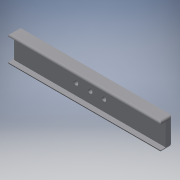
# Autodesk Inventor part: Chain_support
Saved by Autodesk Inventor 2019.3 (Build 233278000, 278)
## iProperties
Created: 2020-09-24
Part Number: Chain_support
Material: Generisch
Document SubType Name: Modeling
Designer: Nicolas Frick
Density: 1 g/cm^3
Appearance: Vorgabe
Author: Nicolas Frick
Autodesk Inventor part; units mm, degrees
ref_plane "YZ Plane" through (0, 0, 0) normal (1, 0, 0) x (0, 1, 0)
ref_plane "XZ Plane" through (0, 0, 0) normal (0, 1, 0) x (-1, 0, 0)
ref_plane "XY Plane" through (0, 0, 0) normal (0, 0, 1) x (1, 0, 0)
sketch "Skizze1" plane through (0, 0, 0) normal (0, 0, 1) x (1, 0, 0)
  line L0 (-23.9848, 119.7892) -> (-23.9848, -119.7892) construction
  line L1 (-23.9848, -119.7892) -> (23.9848, -119.7892) construction
  line L2 (23.9848, -119.7892) -> (23.9848, 119.7892) construction
  line L3 (23.9848, 119.7892) -> (-23.9848, 119.7892) construction
  line L4 (-23.9848, 119.7892) -> (-23.9848, -119.7892) construction
  line L5 (71.859, -124.7444) -> (-78.141, -124.7444)
  line L6 (-78.141, -124.7444) -> (-78.141, -98.7444)
  line L7 (-78.141, -98.7444) -> (71.859, -98.7444)
  line L8 (71.859, -98.7444) -> (71.859, -124.7444)
  circle A0 centre (-16.2025, -111.7444) radius 2.25
  circle A1 centre (11.1538, -111.7444) radius 2.25
  circle A2 centre (-2.2951, -111.7444) radius 2.25
  point P0 (0, 0)
  dimension "d0" = 150
  dimension "d1" = 26
  dimension "d2" = 4.5
  dimension "d3" = 4.5
  dimension "d4" = 4.5
  constraints: 8 end point, 3 centre point, 2 parallel, 1 horizontal, 1 perpendicular
  measures "d0" distance of L6.end L7.end
  measures "d1" distance of L5.end L6.end
  measures "d2" diameter of A0
  measures "d3" diameter of A1
  measures "d4" diameter of A2
ref_plane "Arbeitsebene1" through (175.4546, -108.6892, 6.4137) normal (0, 0, -1) x (0, 1, 0)
extrude "Extrusion1" add sketch "Skizze1" along normal up to surface (6.4137 mm away)
sketch "Skizze3" plane through (-78.141, -124.7444, 6.4137) normal (0, 0, 1) x (1, 0, 0)
  circle A0 centre (75.8459, 13) radius 2.25 construction
  circle A1 centre (89.2948, 13) radius 2.25 construction
  circle A2 centre (61.9385, 13) radius 2.25 construction
  line L0 (0, 26) -> (0, 0) construction
  line L1 (0, 0) -> (150, 0) construction
  line L2 (150, 0) -> (150, 26) construction
  line L3 (150, 26) -> (0, 26) construction
  line L4 (0, 0) -> (0, 26) projected
  line L5 (150, 26) -> (0, 26)
  line L6 (0, 26) -> (0, 24)
  line L7 (0, 24) -> (150, 24)
  line L8 (150, 24) -> (150, 26)
  line L9 (150, 0) -> (0, 0)
  line L10 (0, 0) -> (0, 2)
  line L11 (0, 2) -> (150, 2)
  line L12 (150, 2) -> (150, 0)
  point P0 (78.141, 124.7444)
  dimension "d7" = 2
  dimension "d8" = 2
  constraints: 16 end point, 4 parallel, 2 horizontal, 2 perpendicular, 2 point on line
  measures "d7" distance of L6.end L5.end
  measures "d8" distance of L9.end L10.end
extrude "Extrusion2" add sketch "Skizze3" along normal blind 5
fillet "Rundung1" radius 2 10 edges at (-3.141, -124.7444, 11.4137) (-3.141, -124.7444, 0) (71.859, -111.7444, 0) (-3.141, -98.7444, 11.4137) (71.859, -98.7444, 5.7069) (-78.141, -124.7444, 5.7069) (71.859, -124.7444, 5.7069) (-78.141, -98.7444, 5.7069) (-78.141, -111.7444, 6.4137) (-78.141, -111.7444, 0)
